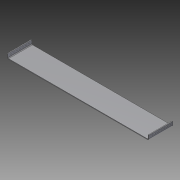
# Autodesk Inventor part: Base Crossbar
Saved by Autodesk Inventor 2012 (Build 160160000, 160)
## iProperties
Created: 2011-10-13
Part Number: Base Crossbar
Material: Default
Document SubType Name: Sheet Metal
Designer: Tushar
Density: 1 g/cm^3
Sheet Metal Rule: Default
Author: Tushar
Autodesk Inventor part; units mm, degrees
ref_plane "YZ Plane" through (0, 0, 0) normal (1, 0, 0) x (0, 1, 0)
ref_plane "XZ Plane" through (0, 0, 0) normal (0, 1, 0) x (-1, 0, 0)
ref_plane "XY Plane" through (0, 0, 0) normal (0, 0, 1) x (1, 0, 0)
sketch "Sketch2" plane through (0, 0, 0) normal (0, 1, 0) x (-1, 0, 0)
  line L0 (-295.529, 50.8) -> (295.529, 50.8)
  line L1 (295.529, 50.8) -> (295.529, -50.8)
  line L2 (295.529, -50.8) -> (-295.529, -50.8)
  line L3 (-295.529, -50.8) -> (-295.529, 50.8)
  point P0 (0, 0)
  dimension "d0" = 295.529
  dimension "d1" = 295.529
  dimension "d2" = 50.8
  dimension "d3" = 50.8
  measures "d0" distance from line of L1 point (0, 0)
  measures "d1" distance from line of point (0, 0) L3
  measures "d2" distance from line of L2 point (0, 0)
  measures "d3" distance from line of L0 point (0, 0)
extrude "Plate1" add sketch "Sketch2" along normal blind 3.048
sketch "Sketch3" plane through (-295.529, 0, 50.8) normal (0, 0, 1) x (1, 0, 0)
  arc A0 (591.058, 0) -> (597.281, 6.223) centre (591.058, 6.223) ccw
  line L0 (591.058, 6.223) -> (597.281, 6.223) construction
  line L1 (591.058, 6.223) -> (591.058, 0) construction
  line L2 (597.281, 6.223) -> (597.281, 19.5834)
  point P0 (591.058, 3.048)
  point P1 (295.529, 0)
  dimension "d5" = 90
  dimension "d6" = 6.223
  dimension "d7" = 6.223
  dimension "d8" = 13.3604
  measures "d5" angle of L1 L0
  measures "d6" radius of A0
  measures "d7" horizontal distance of point (591.058, 3.048) L0.end
  measures "d8" distance of L0.end L2.end
contour flange "Contour Flange1" sketch "Sketch3" thickness 3.048 bend radius 3.048 curves A0 L2 edges at (295.529, 0, 0) running between points at (295.529, 0, -50.8) (295.529, 0, 50.8)
bend "Bend1"
corner "Corner1"
sketch "Sketch4" plane through (-295.529, 0, 50.8) normal (0, 0, 1) x (1, 0, 0)
  arc A0 (-6.223, 6.223) -> (0, 0) centre (0, 6.223) ccw
  line L0 (0, 6.223) -> (-6.223, 6.223) construction
  line L1 (0, 6.223) -> (0, 0) construction
  line L2 (-6.223, 6.223) -> (-6.223, 19.5834)
  point P0 (0, 3.048)
  point P1 (295.529, 0)
  dimension "d18" = 90
  dimension "d19" = 6.223
  dimension "d20" = 6.223
  dimension "d21" = 13.3604
  measures "d18" angle of L0 L1
  measures "d19" radius of A0
  measures "d20" horizontal distance of point (0, 3.048) L0.end
  measures "d21" distance of L0.end L2.end
contour flange "Contour Flange2" sketch "Sketch4" thickness 3.048 bend radius 3.048 curves A0 L2 edges at (-295.529, 0, 0) running between points at (-295.529, 0, 50.8) (-295.529, 0, -50.8)
bend "Bend2"
corner "Corner2"
sketch "Sketch5" plane through (301.752, 6.223, -50.8) normal (1, 0, 0) x (0, 0, -1)
  line L0 (-101.6, 0) -> (-101.6, 13.3604) projected
  line L1 (0, -6.223) -> (-101.6, -6.223) projected
  point P0 (-50.8, -6.223)
  point P1 (-88.9, 6.477)
  dimension "d31" = 12.7
  dimension "d32" = 12.7
  measures "d31" distance from line of L1 point (-88.9, 6.477)
  measures "d32" distance from line of L0 point (-88.9, 6.477)
hole "Hole1" at (301.752, 12.7, 38.1) direction (-1, 0, 0) diameter 3.175 end through all
sketch "Sketch6" plane through (301.752, 6.223, -50.8) normal (1, 0, 0) x (0, 0, -1)
  circle A0 centre (-88.9, 6.477) radius 1.5875 projected
  line L0 (-101.6, 0) -> (-101.6, 13.3604) projected
  line L1 (-88.9, 6.477) -> (-74.5256, 6.477)
  point P0 (-50.8, -6.223)
  constraints: 2 end point, 1 perpendicular
pattern_linear "Rectangular Pattern1" count 7 spacing 12.7 along (0, 0, -1) of "Hole1"
equation "\"d38\" = Thickness"
equation "\"d9\" = BendReliefWidth"
equation "\"d10\" = BendReliefDepth"
equation "\"d11\" = MinimumRemnant"
equation "\"d12\" = BendRadius"
equation "\"d13\" = BendRadius"
equation "\"d15\" = CornerReliefSize"
equation "\"d16\" = GapSize"
equation "\"d17\" = JacobiRadiusSize"
equation "\"d22\" = BendReliefWidth"
equation "\"d23\" = BendReliefDepth"
equation "\"d24\" = MinimumRemnant"
equation "\"d25\" = BendRadius"
equation "\"d26\" = BendRadius"
equation "\"d28\" = CornerReliefSize"
equation "\"d29\" = GapSize"
equation "\"d30\" = JacobiRadiusSize"
equation "\"d1\" = d0"
equation "\"d3\" = d2"
equation "\"BendRadius\" = Thickness"
equation "\"BendReliefWidth\" = Thickness"
equation "\"BendReliefDepth\" = 0.5 * Thickness"
equation "\"CornerReliefSize\" = 4 * Thickness"
equation "\"MinimumRemnant\" = 2 * Thickness"
equation "\"TransitionRadius\" = BendRadius"
equation "\"JacobiRadiusSize\" = BendRadius"
equation "\"GapSize\" = Thickness"
equation "\"d4\" = BendRadius"
equation "\"Thickness\" = 3.048"
body "Solid1"
